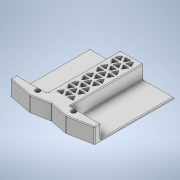
# Autodesk Inventor part: Test1
Saved by Autodesk Inventor 2022 (Build 260153000, 153)
## iProperties
Created: 2022-04-01
Part Number: Test1
Material: Generic
Document SubType Name: Modeling
Designer: thoms
Density: 1 g/cm^3
Appearance: Default
Author: thoms
Autodesk Inventor part; units mm, degrees
ref_plane "YZ Plane" through (0, 0, 0) normal (1, 0, 0) x (0, 1, 0)
ref_plane "XZ Plane" through (0, 0, 0) normal (0, 1, 0) x (-1, 0, 0)
ref_plane "XY Plane" through (0, 0, 0) normal (0, 0, 1) x (1, 0, 0)
sketch "Sketch1" plane through (0, 0, 0) normal (0, 1, 0) x (-1, 0, 0)
  line L0 (27.5, -26) -> (-27.5, -26)
  line L1 (-27.5, -26) -> (-27.5, 26)
  line L2 (-27.5, 26) -> (27.5, 26)
  line L3 (27.5, 26) -> (27.5, -26)
  point P0 (0, 0)
  dimension "d0" = 55
  dimension "d1" = 52
  dimension "d2" = 27.5
  dimension "d3" = 26
  constraints: 8 end point, 2 parallel, 1 horizontal, 1 perpendicular
  measures "d0" distance of L0.start L0.end
  measures "d1" distance of L2.end L0.start
  measures "d2" distance from line of point (0, 0) L3
  measures "d3" distance from line of point (0, 0) L0
extrude "Extrusion1" add sketch "Sketch1" against normal blind 10
sketch "Sketch2" plane through (0, 0, 0) normal (0, 1, 0) x (1, 0, 0)
  line L0 (-27.5, -26) -> (-27.5, 26) projected
  line L1 (-27.5, 26) -> (-7.5, 26)
  line L2 (-7.5, 26) -> (-7.5, -22)
  line L3 (-7.5, -22) -> (-27.5, -22)
  line L4 (-27.5, -22) -> (-27.5, 26)
  line L5 (-27.5, 26) -> (27.5, 26) projected
  line L6 (27.5, 26) -> (7.5, 26)
  line L7 (7.5, 26) -> (7.5, -22)
  line L8 (7.5, -22) -> (27.5, -22)
  line L9 (27.5, -22) -> (27.5, 26)
  line L10 (-27.5, -26) -> (27.5, -26) projected
  point P0 (0, 0)
  dimension "d6" = 15
  dimension "d7" = 7.5
  dimension "d8" = 4
  constraints: 16 end point, 4 parallel, 2 horizontal, 2 perpendicular, 1 point on line
  measures "d6" distance between parallel lines of L7 L2
  measures "d7" distance from line of point (0, 0) L2
  measures "d8" distance between parallel lines of L3 L10
extrude "Extrusion2" cut sketch "Sketch2" against normal blind 9
sketch "Sketch3" plane through (0, 0, 0) normal (0, 1, 0) x (1, 0, 0)
  circle A0 centre (-11.75, -24) radius 1.55
  line L0 (-27.5, -26) -> (27.5, -26) projected
  line L1 (-14.25, 26) -> (14.25, 26)
  line L2 (14.25, 26) -> (14.25, -26)
  line L3 (14.25, -26) -> (-14.25, -26)
  line L4 (-14.25, -26) -> (-14.25, 26)
  line L5 (7.5, 26) -> (-7.5, 26) projected
  circle A1 centre (11.75, -24) radius 1.55
  point P0 (0, 0)
  dimension "d11" = 3.1
  dimension "d12" = 2
  dimension "d13" = 28.5
  dimension "d14" = 14.25
  dimension "d15" = 0
  dimension "d16" = 0
  dimension "d17" = 2.5
  dimension "d18" = 3.1
  dimension "d19" = 2
  dimension "d20" = 2.5
  constraints: 8 end point, 2 centre point, 2 parallel, 1 horizontal, 1 perpendicular
  measures "d11" diameter of A0
  measures "d12" distance from line of L0 A0.centre
  measures "d13" distance of L1.start L1.end
  measures "d14" distance from line of point (0, 0) L4
  measures "d15" distance between parallel lines of L0 L3
  measures "d16" distance between parallel lines of L5 L1
  measures "d17" distance from line of L4 A0.centre
  measures "d18" diameter of A1
  measures "d19" distance from line of L0 A1.centre
  measures "d20" distance from line of L2 A1.centre
extrude "Extrusion3" cut sketch "Sketch3" against normal blind 5 contours A0 | A1
sketch "Sketch4" plane through (0, 0, 0) normal (0, 1, 0) x (1, 0, 0)
  circle A0 centre (-11.75, -24) radius 1.55 projected
  circle A1 centre (11.75, -24) radius 1.55 projected
  line L0 (-11.75, -24) -> (-11.75, -29) construction
  line L1 (-27.5, -22) -> (-27.5, -26) projected
  line L2 (-11.75, -29) -> (-27.5, -26)
  line L3 (11.75, -24) -> (11.75, -29) construction
  line L4 (0, -26.7628) -> (11.75, -29)
  line L5 (-11.75, -29) -> (0, -26.7628)
  line L6 (-27.5, -26) -> (27.5, -26) projected
  line L7 (11.75, -29) -> (27.5, -26)
  line L8 (-27.5, -26) -> (27.5, -26)
  point P0 (0, 0)
  dimension "d25" = 5
  dimension "d26" = 5
  dimension "d29" = 79.22
  dimension "d30" = 79.22
  constraints: 14 end point, 2 vertical, 1 collinear
  measures "d25" distance of L0.start L0.end
  measures "d26" distance of L3.start L3.end
  measures "d29" angle of L3 L4
  measures "d30" angle of L0 L5
extrude "Extrusion4" add sketch "Sketch4" against normal up to surface (10 mm away) contours L2 L6 L7 L4 L5
sketch "Sketch5" plane through (0, 0, 0) normal (0, 1, 0) x (1, 0, 0)
  line L0 (-3.2835, -14.9109) -> (-1.7165, -17.625)
  line L1 (-1.933, -18) -> (-5.067, -18)
  line L2 (-5.2835, -17.625) -> (-3.7165, -14.9109)
  line L3 (-7.5, -22) -> (-27.5, -22) projected
  line L4 (-7.5, 26) -> (-7.5, -22) projected
  line L5 (1.7835, -14.9109) -> (0.2165, -17.625)
  line L6 (-0.2165, -17.625) -> (-1.7835, -14.9109)
  line L7 (-1.567, -14.5359) -> (1.567, -14.5359)
  line L8 (0, -15.8839) -> (0, -17.134) construction
  line L9 (3.2835, -14.9109) -> (1.7165, -17.625)
  line L10 (1.933, -18) -> (5.067, -18)
  line L11 (5.2835, -17.625) -> (3.7165, -14.9109)
  arc A0 (-5.2835, -17.625) -> (-5.067, -18) centre (-5.067, -17.75) ccw
  arc A1 (-3.2835, -14.9109) -> (-3.7165, -14.9109) centre (-3.5, -15.0359) ccw
  arc A2 (-1.933, -18) -> (-1.7165, -17.625) centre (-1.933, -17.75) ccw
  arc A3 (-1.567, -14.5359) -> (-1.7835, -14.9109) centre (-1.567, -14.7859) ccw
  arc A4 (1.7835, -14.9109) -> (1.567, -14.5359) centre (1.567, -14.7859) ccw
  arc A5 (-0.2165, -17.625) -> (0.2165, -17.625) centre (0, -17.5) ccw
  arc A6 (1.7165, -17.625) -> (1.933, -18) centre (1.933, -17.75) ccw
  arc A7 (3.7165, -14.9109) -> (3.2835, -14.9109) centre (3.5, -15.0359) ccw
  arc A8 (5.067, -18) -> (5.2835, -17.625) centre (5.067, -17.75) ccw
  line L12 (-5.067, -13.8864) -> (5.2835, -13.8864) construction
  line L13 (-3.2835, -12.8619) -> (-1.7165, -10.1478)
  line L14 (-1.933, -9.7728) -> (-5.067, -9.7728)
  line L15 (-5.2835, -10.1478) -> (-3.7165, -12.8619)
  line L16 (1.7835, -12.8619) -> (0.2165, -10.1478)
  line L17 (-0.2165, -10.1478) -> (-1.7835, -12.8619)
  line L18 (-1.567, -13.2369) -> (1.567, -13.2369)
  line L19 (0, -11.8889) -> (0, -10.6388) construction
  line L20 (3.2835, -12.8619) -> (1.7165, -10.1478)
  line L21 (1.933, -9.7728) -> (5.067, -9.7728)
  line L22 (5.2835, -10.1478) -> (3.7165, -12.8619)
  arc A9 (-5.067, -9.7728) -> (-5.2835, -10.1478) centre (-5.067, -10.0228) ccw
  arc A10 (-3.7165, -12.8619) -> (-3.2835, -12.8619) centre (-3.5, -12.7369) ccw
  arc A11 (-1.7165, -10.1478) -> (-1.933, -9.7728) centre (-1.933, -10.0228) ccw
  arc A12 (-1.7835, -12.8619) -> (-1.567, -13.2369) centre (-1.567, -12.9869) ccw
  arc A13 (1.567, -13.2369) -> (1.7835, -12.8619) centre (1.567, -12.9869) ccw
  arc A14 (0.2165, -10.1478) -> (-0.2165, -10.1478) centre (0, -10.2728) ccw
  arc A15 (1.933, -9.7728) -> (1.7165, -10.1478) centre (1.933, -10.0228) ccw
  arc A16 (3.2835, -12.8619) -> (3.7165, -12.8619) centre (3.5, -12.7369) ccw
  arc A17 (5.2835, -10.1478) -> (5.067, -9.7728) centre (5.067, -10.0228) ccw
  line L23 (-6.3214, -9.1233) -> (6.5488, -9.1233) construction
  line L24 (-3.2835, -3.3357) -> (-1.7165, -0.6216)
  line L25 (-1.933, -0.2466) -> (-5.067, -0.2466)
  line L26 (-5.2835, -0.6216) -> (-3.7165, -3.3357)
  line L27 (1.7835, -3.3357) -> (0.2165, -0.6216)
  line L28 (-0.2165, -0.6216) -> (-1.7835, -3.3357)
  line L29 (-1.567, -3.7107) -> (1.567, -3.7107)
  line L30 (0, -2.3627) -> (0, -1.1126) construction
  line L31 (3.2835, -3.3357) -> (1.7165, -0.6216)
  line L32 (1.933, -0.2466) -> (5.067, -0.2466)
  line L33 (5.2835, -0.6216) -> (3.7165, -3.3357)
  arc A18 (-5.067, -0.2466) -> (-5.2835, -0.6216) centre (-5.067, -0.4966) ccw
  arc A19 (-3.7165, -3.3357) -> (-3.2835, -3.3357) centre (-3.5, -3.2107) ccw
  arc A20 (-1.7165, -0.6216) -> (-1.933, -0.2466) centre (-1.933, -0.4966) ccw
  arc A21 (-1.7835, -3.3357) -> (-1.567, -3.7107) centre (-1.567, -3.4607) ccw
  arc A22 (1.567, -3.7107) -> (1.7835, -3.3357) centre (1.567, -3.4607) ccw
  arc A23 (0.2165, -0.6216) -> (-0.2165, -0.6216) centre (0, -0.7466) ccw
  arc A24 (1.933, -0.2466) -> (1.7165, -0.6216) centre (1.933, -0.4966) ccw
  arc A25 (3.2835, -3.3357) -> (3.7165, -3.3357) centre (3.5, -3.2107) ccw
  arc A26 (5.2835, -0.6216) -> (5.067, -0.2466) centre (5.067, -0.4966) ccw
  line L34 (-5.067, -4.3602) -> (5.2835, -4.3602) construction
  line L35 (-3.2835, -5.3847) -> (-1.7165, -8.0988)
  line L36 (-1.933, -8.4738) -> (-5.067, -8.4738)
  line L37 (0, -6.3577) -> (0, -7.6078) construction
  arc A27 (-0.2165, -8.0988) -> (0.2165, -8.0988) centre (0, -7.9738) ccw
  line L38 (-1.567, -5.0097) -> (1.567, -5.0097)
  line L39 (1.7835, -5.3847) -> (0.2165, -8.0988)
  line L40 (3.2835, -5.3847) -> (1.7165, -8.0988)
  line L41 (1.933, -8.4738) -> (5.067, -8.4738)
  line L42 (-5.2835, -8.0988) -> (-3.7165, -5.3847)
  line L43 (-0.2165, -8.0988) -> (-1.7835, -5.3847)
  arc A28 (-1.567, -5.0097) -> (-1.7835, -5.3847) centre (-1.567, -5.2597) ccw
  arc A29 (-1.933, -8.4738) -> (-1.7165, -8.0988) centre (-1.933, -8.2238) ccw
  arc A30 (-3.2835, -5.3847) -> (-3.7165, -5.3847) centre (-3.5, -5.5097) ccw
  arc A31 (-5.2835, -8.0988) -> (-5.067, -8.4738) centre (-5.067, -8.2238) ccw
  line L44 (5.2835, -8.0988) -> (3.7165, -5.3847)
  arc A32 (1.7835, -5.3847) -> (1.567, -5.0097) centre (1.567, -5.2597) ccw
  arc A33 (1.7165, -8.0988) -> (1.933, -8.4738) centre (1.933, -8.2238) ccw
  arc A34 (3.7165, -5.3847) -> (3.2835, -5.3847) centre (3.5, -5.5097) ccw
  arc A35 (5.067, -8.4738) -> (5.2835, -8.0988) centre (5.067, -8.2238) ccw
  line L45 (-6.0381, 0.4029) -> (6.5488, 0.4029) construction
  line L46 (-3.2835, 15.7167) -> (-1.7165, 18.4308)
  line L47 (-1.933, 18.8058) -> (-5.067, 18.8058)
  line L48 (-5.2835, 18.4308) -> (-3.7165, 15.7167)
  line L49 (1.7835, 15.7167) -> (0.2165, 18.4308)
  line L50 (-0.2165, 18.4308) -> (-1.7835, 15.7167)
  line L51 (-1.567, 15.3417) -> (1.567, 15.3417)
  line L52 (0, 16.6897) -> (0, 17.9398) construction
  line L53 (3.2835, 15.7167) -> (1.7165, 18.4308)
  line L54 (1.933, 18.8058) -> (5.067, 18.8058)
  line L55 (5.2835, 18.4308) -> (3.7165, 15.7167)
  arc A36 (-5.067, 18.8058) -> (-5.2835, 18.4308) centre (-5.067, 18.5558) ccw
  arc A37 (-3.7165, 15.7167) -> (-3.2835, 15.7167) centre (-3.5, 15.8417) ccw
  arc A38 (-1.7165, 18.4308) -> (-1.933, 18.8058) centre (-1.933, 18.5558) ccw
  arc A39 (-1.7835, 15.7167) -> (-1.567, 15.3417) centre (-1.567, 15.5917) ccw
  arc A40 (1.567, 15.3417) -> (1.7835, 15.7167) centre (1.567, 15.5917) ccw
  arc A41 (0.2165, 18.4308) -> (-0.2165, 18.4308) centre (0, 18.3058) ccw
  arc A42 (1.933, 18.8058) -> (1.7165, 18.4308) centre (1.933, 18.5558) ccw
  arc A43 (3.2835, 15.7167) -> (3.7165, 15.7167) centre (3.5, 15.8417) ccw
  arc A44 (5.2835, 18.4308) -> (5.067, 18.8058) centre (5.067, 18.5558) ccw
  line L56 (-5.067, 14.6922) -> (5.2835, 14.6922) construction
  line L57 (-3.2835, 13.6677) -> (-1.7165, 10.9536)
  line L58 (-1.933, 10.5786) -> (-5.067, 10.5786)
  line L59 (0, 12.6947) -> (0, 11.4446) construction
  arc A45 (-0.2165, 10.9536) -> (0.2165, 10.9536) centre (0, 11.0786) ccw
  line L60 (-1.567, 14.0427) -> (1.567, 14.0427)
  line L61 (1.7835, 13.6677) -> (0.2165, 10.9536)
  line L62 (3.2835, 13.6677) -> (1.7165, 10.9536)
  line L63 (1.933, 10.5786) -> (5.067, 10.5786)
  line L64 (-5.2835, 10.9536) -> (-3.7165, 13.6677)
  line L65 (-0.2165, 10.9536) -> (-1.7835, 13.6677)
  arc A46 (-1.567, 14.0427) -> (-1.7835, 13.6677) centre (-1.567, 13.7927) ccw
  arc A47 (-1.933, 10.5786) -> (-1.7165, 10.9536) centre (-1.933, 10.8286) ccw
  arc A48 (-3.2835, 13.6677) -> (-3.7165, 13.6677) centre (-3.5, 13.5427) ccw
  arc A49 (-5.2835, 10.9536) -> (-5.067, 10.5786) centre (-5.067, 10.8286) ccw
  line L66 (5.2835, 10.9536) -> (3.7165, 13.6677)
  arc A50 (1.7835, 13.6677) -> (1.567, 14.0427) centre (1.567, 13.7927) ccw
  arc A51 (1.7165, 10.9536) -> (1.933, 10.5786) centre (1.933, 10.8286) ccw
  arc A52 (3.7165, 13.6677) -> (3.2835, 13.6677) centre (3.5, 13.5427) ccw
  arc A53 (5.067, 10.5786) -> (5.2835, 10.9536) centre (5.067, 10.8286) ccw
  line L67 (-6.3214, 9.9291) -> (6.5488, 9.9291) construction
  arc A54 (1.7165, 1.4274) -> (1.933, 1.0524) centre (1.933, 1.3024) ccw
  arc A55 (1.7835, 4.1415) -> (1.567, 4.5165) centre (1.567, 4.2665) ccw
  line L68 (3.2835, 4.1415) -> (1.7165, 1.4274)
  arc A56 (3.7165, 4.1415) -> (3.2835, 4.1415) centre (3.5, 4.0165) ccw
  line L69 (1.933, 1.0524) -> (5.067, 1.0524)
  line L70 (5.2835, 1.4274) -> (3.7165, 4.1415)
  arc A57 (5.067, 1.0524) -> (5.2835, 1.4274) centre (5.067, 1.3024) ccw
  line L71 (-1.567, 4.5165) -> (1.567, 4.5165)
  arc A58 (-1.567, 4.5165) -> (-1.7835, 4.1415) centre (-1.567, 4.2665) ccw
  arc A59 (-3.7165, 6.1905) -> (-3.2835, 6.1905) centre (-3.5, 6.3155) ccw
  line L72 (-5.2835, 8.9046) -> (-3.7165, 6.1905)
  arc A60 (-5.067, 9.2796) -> (-5.2835, 8.9046) centre (-5.067, 9.0296) ccw
  line L73 (-3.2835, 6.1905) -> (-1.7165, 8.9046)
  line L74 (-1.933, 9.2796) -> (-5.067, 9.2796)
  arc A61 (-1.7165, 8.9046) -> (-1.933, 9.2796) centre (-1.933, 9.0296) ccw
  line L75 (-5.067, 5.166) -> (5.2835, 5.166) construction
  line L76 (-5.2835, 1.4274) -> (-3.7165, 4.1415)
  arc A62 (-3.2835, 4.1415) -> (-3.7165, 4.1415) centre (-3.5, 4.0165) ccw
  arc A63 (-5.2835, 1.4274) -> (-5.067, 1.0524) centre (-5.067, 1.3024) ccw
  line L77 (-3.2835, 4.1415) -> (-1.7165, 1.4274)
  line L78 (-1.933, 1.0524) -> (-5.067, 1.0524)
  line L79 (1.7835, 4.1415) -> (0.2165, 1.4274)
  line L80 (-0.2165, 1.4274) -> (-1.7835, 4.1415)
  arc A64 (-0.2165, 1.4274) -> (0.2165, 1.4274) centre (0, 1.5524) ccw
  line L81 (0, 3.1685) -> (0, 1.9184) construction
  arc A65 (-1.933, 1.0524) -> (-1.7165, 1.4274) centre (-1.933, 1.3024) ccw
  line L82 (3.2835, 6.1905) -> (1.7165, 8.9046)
  arc A66 (1.567, 5.8155) -> (1.7835, 6.1905) centre (1.567, 6.0655) ccw
  arc A67 (3.2835, 6.1905) -> (3.7165, 6.1905) centre (3.5, 6.3155) ccw
  line L83 (5.2835, 8.9046) -> (3.7165, 6.1905)
  line L84 (1.933, 9.2796) -> (5.067, 9.2796)
  arc A68 (5.2835, 8.9046) -> (5.067, 9.2796) centre (5.067, 9.0296) ccw
  arc A69 (1.933, 9.2796) -> (1.7165, 8.9046) centre (1.933, 9.0296) ccw
  arc A70 (-1.7835, 6.1905) -> (-1.567, 5.8155) centre (-1.567, 6.0655) ccw
  line L85 (-0.2165, 8.9046) -> (-1.7835, 6.1905)
  line L86 (0, 7.1635) -> (0, 8.4136) construction
  arc A71 (0.2165, 8.9046) -> (-0.2165, 8.9046) centre (0, 8.7796) ccw
  line L87 (-1.567, 5.8155) -> (1.567, 5.8155)
  line L88 (1.7835, 6.1905) -> (0.2165, 8.9046)
  line L89 (-6.0381, 19.4553) -> (6.5488, 19.4553) construction
  line L90 (1.7835, 23.1939) -> (0.2165, 20.4798)
  line L91 (-0.2165, 20.4798) -> (-1.7835, 23.1939)
  line L92 (0, 22.2209) -> (0, 20.9708) construction
  arc A72 (-0.2165, 20.4798) -> (0.2165, 20.4798) centre (0, 20.6048) ccw
  arc A73 (-1.933, 20.1048) -> (-1.7165, 20.4798) centre (-1.933, 20.3548) ccw
  line L93 (-1.567, 23.5689) -> (1.567, 23.5689)
  line L94 (-3.2835, 23.1939) -> (-1.7165, 20.4798)
  line L95 (-1.933, 20.1048) -> (-5.067, 20.1048)
  line L96 (-5.2835, 20.4798) -> (-3.7165, 23.1939)
  arc A74 (-5.2835, 20.4798) -> (-5.067, 20.1048) centre (-5.067, 20.3548) ccw
  arc A75 (-3.2835, 23.1939) -> (-3.7165, 23.1939) centre (-3.5, 23.0689) ccw
  arc A76 (-1.567, 23.5689) -> (-1.7835, 23.1939) centre (-1.567, 23.3189) ccw
  arc A77 (1.7165, 20.4798) -> (1.933, 20.1048) centre (1.933, 20.3548) ccw
  arc A78 (1.7835, 23.1939) -> (1.567, 23.5689) centre (1.567, 23.3189) ccw
  arc A79 (3.7165, 23.1939) -> (3.2835, 23.1939) centre (3.5, 23.0689) ccw
  line L97 (1.933, 20.1048) -> (5.067, 20.1048)
  arc A80 (5.067, 20.1048) -> (5.2835, 20.4798) centre (5.067, 20.3548) ccw
  line L98 (5.2835, 20.4798) -> (3.7165, 23.1939)
  line L99 (3.2835, 23.1939) -> (1.7165, 20.4798)
  point P0 (0, 0)
  point P1 (-3.5, -16.8453)
  point P2 (-3.5, -14.5359)
  point P3 (-1.5, -18)
  point P4 (-5.5, -18)
  point P5 (0, -15.6906)
  point P6 (2, -14.5359)
  point P7 (0, -18)
  point P8 (-2, -14.5359)
  point P9 (3.5, -16.8453)
  point P10 (3.5, -14.5359)
  point P11 (1.5, -18)
  point P12 (5.5, -18)
  point P13 (-3.5, -10.9275)
  point P14 (-3.5, -13.2369)
  point P15 (-1.5, -9.7728)
  point P16 (-5.5, -9.7728)
  point P17 (0, -12.0822)
  point P18 (2, -13.2369)
  point P19 (0, -9.7728)
  point P20 (-2, -13.2369)
  point P21 (3.5, -10.9275)
  point P22 (3.5, -13.2369)
  point P23 (1.5, -9.7728)
  point P24 (5.5, -9.7728)
  point P25 (-3.5, -1.4013)
  point P26 (-3.5, -3.7107)
  point P27 (-1.5, -0.2466)
  point P28 (-5.5, -0.2466)
  point P29 (0, -2.556)
  point P30 (2, -3.7107)
  point P31 (0, -0.2466)
  point P32 (-2, -3.7107)
  point P33 (3.5, -1.4013)
  point P34 (3.5, -3.7107)
  point P35 (1.5, -0.2466)
  point P36 (5.5, -0.2466)
  point P37 (-3.5, -7.3191)
  point P38 (-3.5, -5.0097)
  point P39 (-1.5, -8.4738)
  point P40 (0, -6.1644)
  point P41 (2, -5.0097)
  point P42 (0, -8.4738)
  point P43 (-2, -5.0097)
  point P44 (1.5, -8.4738)
  point P45 (3.5, -7.3191)
  point P46 (3.5, -5.0097)
  point P47 (-5.5, -8.4738)
  point P48 (5.5, -8.4738)
  point P49 (-3.5, 17.6511)
  point P50 (-3.5, 15.3417)
  point P51 (-1.5, 18.8058)
  point P52 (-5.5, 18.8058)
  point P53 (0, 16.4964)
  point P54 (2, 15.3417)
  point P55 (0, 18.8058)
  point P56 (-2, 15.3417)
  point P57 (3.5, 17.6511)
  point P58 (3.5, 15.3417)
  point P59 (1.5, 18.8058)
  point P60 (5.5, 18.8058)
  point P61 (-3.5, 11.7333)
  point P62 (-3.5, 14.0427)
  point P63 (-1.5, 10.5786)
  point P64 (0, 12.888)
  point P65 (2, 14.0427)
  point P66 (0, 10.5786)
  point P67 (-2, 14.0427)
  point P68 (1.5, 10.5786)
  point P69 (3.5, 11.7333)
  point P70 (3.5, 14.0427)
  point P71 (-5.5, 10.5786)
  point P72 (5.5, 10.5786)
  point P73 (2, 4.5165)
  point P74 (3.5, 2.2071)
  point P75 (5.5, 1.0524)
  point P76 (-3.5, 4.5165)
  point P77 (-2, 4.5165)
  point P78 (3.5, 4.5165)
  point P79 (-3.5, 8.1249)
  point P80 (-5.5, 9.2796)
  point P81 (-1.5, 9.2796)
  point P82 (-3.5, 2.2071)
  point P83 (-5.5, 1.0524)
  point P84 (-3.5, 5.8155)
  point P85 (-1.5, 1.0524)
  point P86 (0, 3.3618)
  point P87 (0, 1.0524)
  point P88 (1.5, 1.0524)
  point P89 (2, 5.8155)
  point P90 (3.5, 8.1249)
  point P91 (3.5, 5.8155)
  point P92 (5.5, 9.2796)
  point P93 (-2, 5.8155)
  point P94 (0, 9.2796)
  point P95 (0, 6.9702)
  point P96 (1.5, 9.2796)
  point P97 (-1.5, 20.1048)
  point P98 (0, 22.4142)
  point P99 (0, 20.1048)
  point P100 (1.5, 20.1048)
  point P101 (-3.5, 23.5689)
  point P102 (-2, 23.5689)
  point P103 (-3.5, 21.2595)
  point P104 (-5.5, 20.1048)
  point P105 (2, 23.5689)
  point P106 (3.5, 21.2595)
  point P107 (3.5, 23.5689)
  point P108 (5.5, 20.1048)
  dimension "d33" = 4
  dimension "d35" = 4
  dimension "d36" = 4
  dimension "d37" = 4
  dimension "d39" = 0
  dimension "d40" = 0
  dimension "d41" = 0.25
  dimension "d42" = 0.6495
  dimension "d43" = 0.6495
  dimension "d44" = 0.6495
  dimension "d45" = 0.6495
  constraints: 340 symmetric about line, 196 end point, 162 point on circle, 162 point on line, 81 centre point, 18 tangent, 8 equal radius, 4 horizontal, 1 vertical, 86 other
  measures "d33" distance of point (-5.5, -18) point (-3.5, -14.536)
  measures "d35" distance between parallel lines of L3 L1
  measures "d36" distance from line of L4 point (-3.5, -16.845)
  measures "d37" distance of point (-2, -14.536) point (2, -14.536)
  measures "d39" distance from line of L1 point (0, -18)
  measures "d40" horizontal distance of point (0, 0) point (0, -15.691)
  measures "d41" radius of A0
  measures "d42" distance between parallel lines of L7 L12
  measures "d43" distance between parallel lines of L21 L23
  measures "d44" distance between parallel lines of L32 L45
  measures "d45" distance between parallel lines of L89 L54
extrude "Extrusion5" cut sketch "Sketch5" against normal up to surface (10 mm away)
fillet "Fillet1" radius 0.5 30 edges at (-19.625, 0, 27.5) (-5.875, 0, 27.8814) (5.875, 0, 27.8814) (19.625, 0, 27.5) (27.5, 0, 24) (17.5, 0, 22) (7.5, 0, -2) (0, 0, -26) (-7.5, 0, -2) (-17.5, 0, 22) (-27.5, 0, 24) (-27.5, -5, 26) (-27.5, -4.5, 22) (-11.75, -5, 29) (0, -5, 26.7628) (11.75, -5, 29) (27.5, -5, 26) (27.5, -4.5, 22) (7.5, -4.5, 22) (7.5, -4.5, -26) (-7.5, -4.5, -26) (-7.5, -4.5, 22) (-27.5, -9, -2) (-17.5, -9, -26) (17.5, -9, -26) (27.5, -9, -2) (17.5, -9, 22) (-17.5, -9, 22) (-7.5, -9, -2) (7.5, -9, -2)
body "Solid1"
